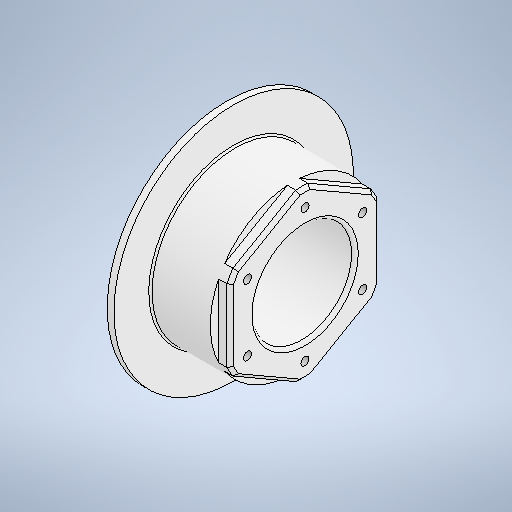
# Autodesk Inventor part: joint4_axis3
Saved by Autodesk Inventor 2025.3 (Build 293356030, 356C)
## iProperties
Created: 2025-10-28
Part Number: joint4_axis3
Material: PLA filament
Document SubType Name: Modeling
Designer: MSI
Density: 1.2 g/cm^3
Appearance: 일반
Mass: 45.6575 g
Surface Area: 146.46 cm^2
Volume: 38.0479 cm^3
Author: MSI
Autodesk Inventor part; units mm, degrees
ref_plane "YZ Plane" through (0, 0, 0) normal (1, 0, 0) x (0, 1, 0)
ref_plane "XZ Plane" through (0, 0, 0) normal (0, 1, 0) x (-1, 0, 0)
ref_plane "XY Plane" through (0, 0, 0) normal (0, 0, 1) x (1, 0, 0)
sketch "스케치1" plane through (0, 0, 0) normal (0, 0, 1) x (1, 0, 0)
  line L0 (0, 0) -> (29.5, 0)
  line L1 (29.5, 0) -> (29.5, 25)
  line L2 (29.5, 25) -> (0, 25)
  line L3 (0, 25) -> (0, 0)
  line L4 (6, 0) -> (8, 0)
  line L5 (8, 0) -> (8, 36)
  line L6 (8, 36) -> (6, 36)
  line L7 (6, 36) -> (6, 0)
  point P0 (7, 36)
  point P1 (6, 25)
  point P2 (8, 25)
  dimension "d3" = 50
  dimension "d12" = 29.5
  dimension "d70" = 6
  dimension "d71" = 2
  dimension "d72" = 72
  constraints: 16 end point, 4 parallel, 2 horizontal, 2 perpendicular, 1 midpoint, 1 point on line
  measures "d3" diameter of L2 L0
  measures "d12" distance of L1.end L2.end
  measures "d70" distance between parallel lines of L7 L3
  measures "d71" distance of L5.end L6.end
  measures "d72" diameter of point (7, 36) L0
revolve "회전1" add sketch "스케치1" angle 360 about axis through (0, 0, 0) along (1, 0, 0)
sketch "스케치3" plane through (29.5, 0, 0) normal (1, 0, 0) x (0, 0, -1)
  circle A0 centre (0, 0) radius 25 projected
  constraints: 1 coincident
hole "구멍2" at (29.5, 0, 0) direction (-1, 0, 0) diameter 30 end through all
chamfer "모따기1" distance 5 angle 30 1 edges at (0, -25, 0) measured on face at (0, -24.5, 0)
sketch "스케치4" plane through (0, 0, 0) normal (-1, 0, 0) x (0, 0, 1)
  circle A0 centre (0, 0) radius 25 projected
  line L0 (0, 25.9808) -> (22.5, 12.9904)
  line L1 (22.5, 12.9904) -> (22.5, -12.9904)
  line L2 (22.5, -12.9904) -> (0, -25.9808)
  line L3 (0, -25.9808) -> (-22.5, -12.9904)
  line L4 (-22.5, -12.9904) -> (-22.5, 12.9904)
  line L5 (-22.5, 12.9904) -> (0, 25.9808)
  point P0 (1.8127, 24.9342)
  point P1 (20.6873, 14.0369)
  point P2 (22.5, 10.8972)
  point P3 (22.5, -10.8972)
  point P4 (20.6873, -14.0369)
  point P5 (1.8127, -24.9342)
  point P6 (-1.8127, -24.9342)
  point P7 (-20.6873, -14.0369)
  point P8 (-22.5, -10.8972)
  point P9 (-22.5, 10.8972)
  point P10 (-20.6873, 14.0369)
  point P11 (-1.8127, 24.9342)
  dimension "d27" = 45
  constraints: 12 end point, 1 coincident, 1 vertical alignment, 13 other
  measures "d27" distance between parallel lines of L1 L4
extrude "돌출1" cut sketch "스케치4" against normal blind 6 contours A0 L1 | L0 A0 | A0 L2 | L5 A0 | A0 L3 | L4 A0
sketch "스케치8" plane through (0, 0, 0) normal (-1, 0, 0) x (0, 0, 1)
  line L0 (0, 0) -> (0, 20)
  dimension "d45" = 20
  constraints: 2 end point, 1 vertical
  measures "d45" distance of L0.start L0.end
hole "구멍4" at (0, 20, 0) direction (1, 0, 0) diameter 2.459 depth 8.8 tip angle 118 thread size "M3x0.5" class "6H" standard "ISO Metric profile"
pattern_circular "원형 패턴2" count 6 over 360 about axis through (-76.5106, 0, 0) along (1, 0, 0) of "구멍4"
sketch "스케치6" plane through (29.5, 0, 0) normal (1, 0, 0) x (0, 0, -1)
  line L0 (0, 25.9808) -> (22.5, 12.9904)
  line L1 (22.5, 12.9904) -> (22.5, -12.9904)
  line L2 (22.5, -12.9904) -> (0, -25.9808)
  line L3 (0, -25.9808) -> (-22.5, -12.9904)
  line L4 (-22.5, -12.9904) -> (-22.5, 12.9904)
  line L5 (-22.5, 12.9904) -> (0, 25.9808)
  circle A0 centre (0, 0) radius 25 projected
  point P0 (1.8127, -24.9342)
  point P1 (20.6873, -14.0369)
  point P2 (-20.6873, -14.0369)
  point P3 (-1.8127, -24.9342)
  point P4 (22.5, 10.8972)
  point P5 (22.5, -10.8972)
  point P6 (-22.5, 10.8972)
  point P7 (-22.5, -10.8972)
  point P8 (20.6873, 14.0369)
  point P9 (1.8127, 24.9342)
  point P10 (-1.8127, 24.9342)
  point P11 (-20.6873, 14.0369)
  dimension "d28" = 45
  constraints: 12 end point, 1 coincident, 1 vertical alignment, 13 other
  measures "d28" distance between parallel lines of L1 L4
extrude "돌출2" cut sketch "스케치6" against normal blind 3.5 contours L0 A0 L5 | A0 L0 | L5 A0 | L0 L1 A0 | A0 L4 L5 | A0 L1 | L4 A0 | L1 L2 A0 | A0 L3 L4 | A0 L2 | L3 A0 | L2 L3 A0
sketch "스케치9" plane through (29.5, -10.8972, -22.5) normal (1, 0, 0) x (0, 0, -1)
  line L0 (-22.5, 10.8972) -> (-22.5, 30.8972)
  dimension "d56" = 20
  constraints: 2 end point, 1 vertical
  measures "d56" distance of L0.start L0.end
hole "구멍5" at (29.5, 20, 0) direction (-1, 0, 0) diameter 2.459 depth 8.8 tip angle 118 thread size "M3x0.5" class "6H" standard "ISO Metric profile"
pattern_circular "원형 패턴3" count 6 over 360 about axis through (-76.5106, 0, 0) along (1, 0, 0) of "구멍5"
chamfer "모따기3" distance 1 angle 45 13 edges at (29.5, 0, 22.5) (29.5, 12.5, 21.6506) (29.5, 19.4856, 11.25) (29.5, 24.9835, 0.907) (29.5, 24.9835, -0.907) (29.5, 19.4856, -11.25) (29.5, 12.5, -21.6506) (29.5, -12.5, -21.6506) (29.5, 0, -22.5) (29.5, -19.4856, -11.25) (29.5, -25, 0) (29.5, -19.4856, 11.25) (29.5, -12.5, 21.6506)
fillet "모깎기1" radius 0.5 1 edges at (8, -25, 0)
fillet "모깎기2" radius 1 1 edges at (29.5, 0, 15)
equation "\"d3\" = joint4_axis3_d2"
equation "\"d13\" = joint4_axis3_d1"
equation "\"joint4_belt_centor\" = 157.367"
equation "\"joint4_axis2_L\" = 58.803"
equation "\"joint4_axis2_b1\" = 35"
equation "\"joint4_axis2_d\" = 19"
equation "\"joint4_miter_m\" = 2"
equation "\"joint4_miter_a\" = 20deg"
equation "\"joint4_miter_z\" = 79"
equation "\"joint4_miter_b\" = 6.90139"
equation "\"joint4_axis3_L\" = 23.5"
equation "\"joint4_axis3_d1\" = 30"
equation "\"joint4_axis3_d2\" = 50"
equation "\"joint3_belt_centor\" = 157.367"
equation "\"joint3_axis2_L\" = 16"
equation "\"joint3_axis2_d\" = 19"
equation "\"joint3_planetary_m\" = 1.5"
equation "\"joint3_planetary_a\" = 20deg"
equation "\"joint3_planetary_np\" = 4"
equation "\"joint3_sun_z\" = 18"
equation "\"joint3_sun_b\" = 17"
equation "\"joint3_planet_z\" = 36"
equation "\"joint3_planet_b\" = 17"
equation "\"joint3_ring_b\" = 9"
equation "\"joint3_axis3_d\" = 29"
equation "\"joint3_miter_m\" = 5.5"
equation "\"joint3_miter_a\" = 20deg"
equation "\"joint3_miter_z\" = 28"
equation "\"joint3_miter_b\" = 13.65957"
equation "\"joint3_axis4_L\" = 23.5"
